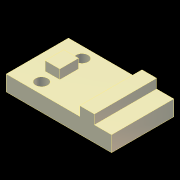
# Autodesk Inventor part: Lift Spacer
Saved by Autodesk Inventor 2015 SP1 (Build 190203100, 203)
## iProperties
Created: 2014-09-14
Part Number: Lift Spacer
Document SubType Name: Modeling
Designer: Family Room
Density: 1 g/cm^3
Material: Generic
Appearance: Nylon 6
Author: Family Room
Autodesk Inventor part; units mm, degrees
ref_plane "YZ Plane" through (0, 0, 0) normal (1, 0, 0) x (0, 1, 0)
ref_plane "XZ Plane" through (0, 0, 0) normal (0, 1, 0) x (-1, 0, 0)
ref_plane "XY Plane" through (0, 0, 0) normal (0, 0, 1) x (1, 0, 0)
sketch "Sketch1" plane through (0, 0, 0) normal (0, 0, 1) x (1, 0, 0)
  line L0 (-21.4986, 0) -> (21.4986, 0)
  line L1 (21.4986, 0) -> (21.4986, 6.35)
  line L2 (-21.4986, 6.35) -> (-21.4986, 0)
  line L3 (-8.524, 6.35) -> (-8.524, 10.16)
  line L4 (-8.524, 10.16) -> (-14.4986, 10.16)
  line L5 (-14.4986, 6.35) -> (-21.4986, 6.35)
  line L6 (14.4986, 6.35) -> (14.4986, 10.16)
  line L7 (14.4986, 10.16) -> (8.524, 10.16)
  line L8 (8.524, 10.16) -> (8.524, 6.35)
  line L9 (21.4986, 6.35) -> (14.4986, 6.35)
  line L10 (8.524, 6.35) -> (-8.524, 6.35)
  line L11 (-14.4986, 10.16) -> (-14.4986, 6.35)
  point P0 (0, 0)
  point P1 (0, 0)
  point P2 (0, 6.35)
  dimension "d0" = 42.9972
  dimension "d1" = 6.35
  dimension "d5" = 5.9746
  dimension "d13" = 7
  dimension "d30" = 3.81
  dimension "d31" = 17.048
  constraints: 24 end point, 5 collinear, 5 horizontal, 5 vertical, 2 midpoint, 1 coincident, 1 vertical alignment
  measures "d0" distance of L2.start L1.end
  measures "d1" distance of L1.end L0.end
  measures "d5" distance of L7.end L6.end
  measures "d13" distance of L1.end L6.start
  measures "d30" distance between parallel lines of L7 L9
  measures "d31" distance between parallel lines of L8 L3
extrude "Extrusion1" add sketch "Sketch1" along normal blind 25.4
sketch "Sketch2" plane through (-14.4986, 6.35, 0) normal (-1, 0, 0) x (0, 0, 1)
  line L0 (0, 3.81) -> (25.4, 3.81) projected
  line L1 (0, 0) -> (25.4, 0) projected
  line L2 (0, 0) -> (8.89, 0)
  line L3 (8.89, 0) -> (8.89, 3.81)
  line L4 (8.89, 3.81) -> (0, 3.81)
  line L5 (0, 3.81) -> (0, 0)
  line L6 (25.4, 0) -> (16.51, 0)
  line L7 (16.51, 0) -> (16.51, 3.81)
  line L8 (16.51, 3.81) -> (25.4, 3.81)
  line L9 (25.4, 3.81) -> (25.4, 0)
  dimension "d32" = 8.89
  constraints: 16 end point, 4 parallel, 2 horizontal, 2 perpendicular, 2 point on line, 1 collinear
  measures "d32" distance between parallel lines of L9 L7
extrude "Extrusion2" cut sketch "Sketch2" against normal blind 15.24 contours L0 L3 L1 L5 | L0 L9 L1 L7
sketch "Sketch3" plane through (-21.4986, 6.35, 25.4) normal (0, 1, 0) x (1, 0, 0)
  line L0 (0, 0) -> (9.9964, 0)
  line L1 (0, 0) -> (30.0226, 0) projected
  line L2 (9.9964, 0) -> (9.9964, 4.445)
  line L3 (9.9964, 0) -> (9.9964, 4.445)
  line L4 (0, 25.4) -> (42.9972, 25.4) projected
  line L5 (9.9964, 25.4) -> (5.5514, 25.4)
  line L6 (9.9964, 25.4) -> (9.9964, 20.955)
  point P0 (21.4986, 25.4)
  dimension "d20" = 4.445
  dimension "d21" = 4.445
  constraints: 10 end point, 3 point on line, 2 perpendicular, 1 collinear
  measures "d20" distance of L5.start L6.end
  measures "d21" distance of L0.end L2.end
hole "Hole1" at (-11.5022, 6.35, 20.955) at (-11.5022, 6.35, 4.445) direction (0, -1, 0) diameter 4.953 end through all
body "Solid1"
